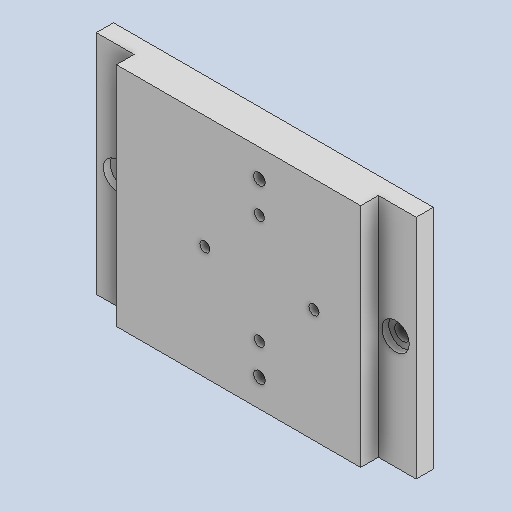
# Autodesk Inventor part: aom mount
Saved by Autodesk Inventor 2024.2 (Build 282272000, 272)
## iProperties
Created: 2021-02-11
Part Number: aom mount
Material: Generic
Document SubType Name: Modeling
Designer: maria
Density: 1 g/cm^3
Appearance: Default
Author: maria
Autodesk Inventor part; units mm, degrees
ref_plane "YZ Plane" through (0, 0, 0) normal (1, 0, 0) x (0, 1, 0)
ref_plane "XZ Plane" through (0, 0, 0) normal (0, 1, 0) x (-1, 0, 0)
ref_plane "XY Plane" through (0, 0, 0) normal (0, 0, 1) x (1, 0, 0)
sketch "Sketch1" plane through (0, 0, 0) normal (0, 0, 1) x (1, 0, 0)
  line L0 (-35.55, -33) -> (35.55, -33)
  line L1 (35.55, -33) -> (35.55, 33)
  line L2 (35.55, 33) -> (-35.55, 33)
  line L3 (-35.55, 33) -> (-35.55, -33)
  line L4 (-35.55, -33) -> (35.55, 33) construction
  line L5 (35.55, -33) -> (-35.55, 33) construction
  point P0 (0, 0)
  dimension "LENGTH" = 71.1
  dimension "WIDTH" = 66
  constraints: 12 end point, 2 midpoint, 2 parallel, 1 horizontal, 1 perpendicular
  measures "LENGTH" distance of L1.end L2.end
  measures "WIDTH" distance of L2.end L0.start
extrude "Extrusion1" add sketch "Sketch1" along normal blind 10.16
sketch "Sketch2" plane through (0, 0, 0) normal (0, 0, 1) x (1, 0, 0)
  line L0 (46.55, -33) -> (-46.55, -33)
  line L1 (-46.55, -33) -> (-46.55, 33)
  line L2 (-46.55, 33) -> (46.55, 33)
  line L3 (46.55, 33) -> (46.55, -33)
  line L4 (46.55, -33) -> (-46.55, 33) construction
  line L5 (-46.55, -33) -> (46.55, 33) construction
  point P0 (0, 0)
  dimension "d4" = 93.1
  dimension "d5" = 66
  constraints: 12 end point, 2 midpoint, 2 parallel, 1 horizontal, 1 perpendicular
  measures "d4" distance of L1.end L2.end
  measures "d5" distance of L2.end L0.start
extrude "Extrusion2" add sketch "Sketch2" along normal blind 5
sketch "Sketch3" plane through (0, 0, 5) normal (0, 0, 1) x (1, 0, 0)
  line L0 (-46.55, 33) -> (-46.55, -33) projected
  line L1 (46.55, -33) -> (46.55, 33) projected
  point P0 (0, 0)
  point P1 (-40.55, 0)
  point P2 (40.55, 0)
  dimension "d8" = 6
  dimension "d9" = 6
  dimension "d10" = 0
  dimension "d11" = 0
  measures "d8" distance from line of L0 point (-40.55, 0)
  measures "d9" distance from line of L1 point (40.55, 0)
  measures "d10" vertical distance of point (0, 0) point (-40.55, 0)
  measures "d11" vertical distance of point (40.55, 0) point (0, 0)
hole "Hole1" at (40.55, 0, 5) at (-40.55, 0, 5) direction (0, 0, -1) diameter 4.5 end through all counterbore diameter 8 counterbore depth 2 clearance for "Socket Head Cap Screw" size "#8" standard "Ansi Unified Screw Threads"
sketch "Sketch4" plane through (0, 0, 0) normal (0, 0, -1) x (-1, 0, 0)
  line L0 (-35.55, -33) -> (-35.55, 33) projected
  point P0 (0, 0)
  point P1 (-6.09, -25)
  point P2 (-6.09, 24.99)
  dimension "d19" = 25
  dimension "d20" = 49.99
  dimension "d21" = 29.46
  dimension "d22" = 29.46
  measures "d19" vertical distance of point (0, 0) point (-6.09, -25)
  measures "d20" distance of point (-6.09, 24.99) point (-6.09, -25)
  measures "d21" distance from line of point (-6.09, -25) L0
  measures "d22" distance from line of L0 point (-6.09, 24.99)
hole "Hole2" at (6.09, -25, 0) at (6.09, 24.99, 0) direction (0, 0, 1) diameter 3.4 end through all counterbore diameter 6.5 counterbore depth 3 clearance for "Socket Head Cap Screw" size "M3" standard "Ansi Metric M Profile"
sketch "Sketch5" plane through (0, 0, 0) normal (0, 0, -1) x (-1, 0, 0)
  circle A0 centre (-6.09, 0) radius 15.875
  point P0 (0, 0)
  point P1 (-6.09, -15.875)
  point P2 (9.785, 0)
  point P3 (-6.09, 15.875)
  point P4 (-21.965, 0)
  dimension "d32" = 6.09
  dimension "d33" = 0
  dimension "d34" = 31.75
  constraints: 4 point on circle, 1 centre point
  measures "d32" distance of point (0, 0) A0.centre
  measures "d33" vertical distance of point (0, 0) A0.centre
  measures "d34" diameter of A0
hole "Hole3" at (6.09, -15.875, 0) at (-9.785, 0, 0) at (6.09, 15.875, 0) at (21.965, 0, 0) direction (0, 0, 1) diameter 2.946 end through all counterbore diameter 5.558 counterbore depth 2.845 clearance for "Socket Head Cap Screw" size "#4" standard "Ansi Unified Screw Threads"
equation "\"d5\" = WIDTH"
body "Solid1"
